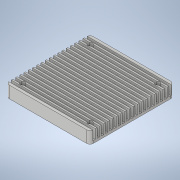
# Autodesk Inventor part: 20_Cube_Sampleholder
Saved by Autodesk Inventor 2022 (Build 260153000, 153)
## iProperties
Created: 2018-07-23
Part Number: 20_Cube_Sampleholder
Material: Generisch
Document SubType Name: Modeling
Designer: diederichbenedict
Density: 1 g/cm^3
Appearance: Vorgabe
Author: diederichbenedict
Autodesk Inventor part; units mm, degrees
ref_plane "YZ Plane" through (0, 0, 0) normal (1, 0, 0) x (0, 1, 0)
ref_plane "XZ Plane" through (0, 0, 0) normal (0, 1, 0) x (-1, 0, 0)
ref_plane "Arbeitsebene1" through (0, 0, 0) normal (0, 0, 1) x (1, 0, 0)
sketch "Skizze1" plane through (0, 0, 0) normal (0, 0, 1) x (1, 0, 0)
  arc A0 (-22.9, 24.9) -> (-24.9, 22.9) centre (-22.9, 22.9) ccw projected
  line L0 (-24.9, 22.9) -> (-24.9, -22.9) projected
  arc A1 (-24.9, -22.9) -> (-22.9, -24.9) centre (-22.9, -22.9) ccw projected
  line L1 (-22.9, -24.9) -> (22.9, -24.9) projected
  arc A2 (22.9, -24.9) -> (24.9, -22.9) centre (22.9, -22.9) ccw projected
  line L2 (24.9, -22.9) -> (24.9, 22.9) projected
  arc A3 (24.9, 22.9) -> (22.9, 24.9) centre (22.9, 22.9) ccw projected
  line L3 (22.9, 24.9) -> (-22.9, 24.9) projected
  circle A4 centre (20, 20) radius 1.6 projected
  circle A5 centre (-20, -20) radius 1.6 projected
  circle A6 centre (20, -20) radius 1.6 projected
  circle A7 centre (-20, 20) radius 1.6 projected
  arc A8 (6.7383, -21.066) -> (8.3017, -21.066) centre (7.52, -20.62) ccw projected
  line L4 (6.7383, -21.066) -> (-6.9383, -21.066) projected
  arc A9 (-8.5017, -21.066) -> (-6.9383, -21.066) centre (-7.72, -20.62) ccw projected
  line L5 (-8.5017, -21.066) -> (-17.9, -21.066) projected
  line L6 (-17.9, -21.066) -> (-17.9, 21.066) projected
  line L7 (-17.9, 21.066) -> (17.9, 21.066) projected
  line L8 (17.9, 21.066) -> (17.9, 12) projected
  arc A10 (14.9, 9) -> (17.9, 12) centre (14.9, 12) ccw projected
  line L9 (14.5, 9) -> (14.9, 9) projected
  arc A11 (14.5, 9) -> (11.5, 6) centre (14.5, 6) ccw projected
  line L10 (11.5, -6) -> (11.5, 6) projected
  arc A12 (11.5, -6) -> (14.5, -9) centre (14.5, -6) ccw projected
  line L11 (14.9, -9) -> (14.5, -9) projected
  arc A13 (17.9, -12) -> (14.9, -9) centre (14.9, -12) ccw projected
  line L12 (17.9, -12) -> (17.9, -21.066) projected
  line L13 (17.9, -21.066) -> (8.3017, -21.066) projected
  arc A14 (13.4381, 5.6873) -> (13.3881, 5.2) centre (15.7881, 5.2) ccw projected
  line L14 (13.4381, 5.6873) -> (13.4381, 7.6) projected
  line L15 (13.4381, 7.6) -> (15.7881, 7.6) projected
  arc A15 (18.1881, 5.2) -> (15.7881, 7.6) centre (15.7881, 5.2) ccw projected
  line L16 (18.1881, 5.2) -> (18.1881, -5.2) projected
  arc A16 (15.7881, -7.6) -> (18.1881, -5.2) centre (15.7881, -5.2) ccw projected
  line L17 (15.7881, -7.6) -> (13.4381, -7.6) projected
  line L18 (13.4381, -7.6) -> (13.4381, -5.6873) projected
  arc A17 (13.3881, -5.2) -> (13.4381, -5.6873) centre (15.7881, -5.2) ccw projected
  line L19 (13.3881, -5.2) -> (13.3881, 5.2) projected
  line L20 (17.9, 21.066) -> (17.9, -21.066)
  point P0 (0, 0)
  constraints: 2 end point, 1 vertical
extrude "Extrusion1" add sketch "Skizze1" along normal blind 7 contours L3 A3 L2 A2 L1 A1 L0 A0 | A4 | A5 | A6 | A7 | L4 A9 L5 L6 L7 L8 A10 L9 A11 L10 A12 L11 A13 L12 L13 A8 | A13 L11 A12 L10 A11 L9 A10 L20 A15 L15 L14 A14 L19 A17 L18 L17 A16 | L20 A15 L16 A16 | A16 L17 L18 A17 L19 A14 L14 L15 A15 L20
sketch "Skizze2" plane through (0, 0, 7) normal (0, 0, 1) x (1, 0, 0)
  circle A0 centre (-20, 20) radius 1.6 projected
  circle A1 centre (20, 20) radius 1.6 projected
  circle A2 centre (20, -20) radius 1.6 projected
  circle A3 centre (-20, -20) radius 1.6 projected
  line L0 (24.9, -22.9) -> (24.9, 22.9) projected
  line L1 (-24.9, 0.75) -> (24.9, 0.75)
  line L2 (24.9, 0.75) -> (24.9, -0.75)
  line L3 (24.9, -0.75) -> (-24.9, -0.75)
  line L4 (-24.9, -0.75) -> (-24.9, 0.75)
  line L5 (-24.9, 0.75) -> (24.9, -0.75) construction
  line L6 (24.9, 0.75) -> (-24.9, -0.75) construction
  point P0 (0, 0)
  dimension "d2" = 1.5
  constraints: 12 end point, 2 midpoint, 2 parallel, 1 horizontal, 1 perpendicular, 1 point on line
  measures "d2" distance of L1.end L2.end
extrude "Extrusion2" cut sketch "Skizze2" against normal blind 5.5 contours L3 L4 L1 L0
pattern_linear "Rechteckige Anordnung1" count 10 spacing 2.5 along (0, -1, 0) count 10 spacing 2.5 along (0, 1, 0) of "Extrusion2"
sketch "Skizze3" plane through (0, 0, 7) normal (0, 0, 1) x (1, 0, 0)
  circle A0 centre (-20, -20) radius 1.6 projected
  line L0 (18.8686, -21.1314) -> (18.4, -21.6) projected
  arc A1 (22.9, -19.2319) -> (19.2319, -22.9) centre (20, -20) ccw projected
  circle A2 centre (20, 20) radius 1.6 projected
  circle A3 centre (-20, 20) radius 1.6 projected
  point P0 (0, 0)
hole "Bohrung1" at (-20, 20, 7) at (20, 20, 7) at (20, -20, 7) at (-20, -20, 7) direction (0, 0, -1) diameter 2.7 end through all
